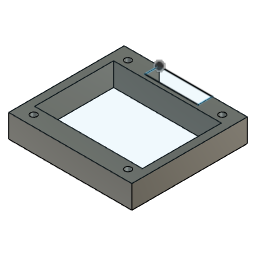
OLEDHolder (Autodesk Fusion 360 design; units mm, degrees)
Autodesk Fusion 360 part; units mm, degrees
sketch "Sketch1" plane through (0, 0, 0) normal (0, 0, 1) x (1, 0, 0)
  line L0 (16, 15) -> (-16, 15)
  line L1 (-16, 15) -> (-16, -15)
  line L2 (-16, -15) -> (16, -15)
  line L3 (16, -15) -> (16, 15)
  line L4 (16, 15) -> (-16, -15) construction
  line L5 (-16, 15) -> (16, -15) construction
  line L6 (14, 10.25) -> (-14, 10.25)
  line L7 (-14, 10.25) -> (-14, -10.25)
  line L8 (-14, -10.25) -> (14, -10.25)
  line L9 (14, -10.25) -> (14, 10.25)
  line L10 (14, 10.25) -> (-14, -10.25) construction
  line L11 (-14, 10.25) -> (14, -10.25) construction
  dimension "d1" = 32
  dimension "d2" = 30
  dimension "d3" = 28
  dimension "d4" = 20.5
  constraint horizontal L0
  constraint perpendicular L0 L1
  constraint parallel L0 L2
  constraint parallel L1 L3
  constraint coincident L4 origin
  constraint coincident L5 origin
  constraint horizontal L6
  constraint perpendicular L6 L7
  constraint parallel L6 L8
  constraint parallel L7 L9
  constraint coincident L10 origin
  constraint coincident L11 origin
  measures "d1" distance of L1.end L2.end
  measures "d2" distance of L0.end L1.end
  measures "d3" distance of L7.end L8.end
  measures "d4" distance of L6.end L7.end
extrude "Extrude1" add sketch "Sketch1" along normal blind 6
sketch "Sketch2" plane through (0, 0, 6) normal (0, 0, 1) x (-1, 0, 0)
  line L0 (-14, -10.25) -> (-14, 10.25)
  line L1 (-14, 10.25) -> (14, 10.25)
  line L2 (14, 10.25) -> (14, -10.25)
  line L3 (14, -10.25) -> (-14, -10.25)
  line L4 (-16, 15) -> (-16, -15)
  line L5 (-16, -15) -> (16, -15)
  line L6 (16, -15) -> (16, 15)
  line L7 (16, 15) -> (-16, 15)
  line L8 (6.895, -15) -> (-6.895, -15)
  line L9 (-6.895, -15) -> (-6.895, -11.3)
  line L10 (-6.895, -11.3) -> (6.895, -11.3)
  line L11 (6.895, -11.3) -> (6.895, -15)
  dimension "d7" = 13.79
  dimension "d8" = 3.7
  constraint horizontal L8
  constraint vertical L9
  constraint horizontal L10
  constraint vertical L11
  constraint coincident L5 L8.start
  measures "d7" distance of L8.start L8.end
  measures "d8" distance of L8.start L10.end
extrude "Extrude2" cut sketch "Sketch2" against normal blind 5 contours L5 L8 L9 L10 L11
sketch "Sketch3" plane through (0, 0, 6) normal (0, 0, 1) x (-1, 0, 0)
  line L0 (6.895, -11.3) -> (6.895, -15)
  line L1 (6.895, -15) -> (16, -15)
  line L2 (16, -15) -> (16, 15)
  line L3 (16, 15) -> (-16, 15)
  line L4 (-16, 15) -> (-16, -15)
  line L5 (-16, -15) -> (-6.895, -15)
  line L6 (-6.895, -15) -> (-6.895, -11.3)
  line L7 (-6.895, -11.3) -> (6.895, -11.3)
  line L8 (-14, -10.25) -> (-14, 10.25)
  line L9 (-14, 10.25) -> (14, 10.25)
  line L10 (14, 10.25) -> (14, -10.25)
  line L11 (14, -10.25) -> (-14, -10.25)
  line L12 (-13.75, -13.75) -> (13.75, -13.75)
  line L13 (13.75, -13.75) -> (13.75, 13.75)
  line L14 (13.75, 13.75) -> (-13.75, 13.75)
  line L15 (-13.75, 13.75) -> (-13.75, -13.75)
  line L16 (-13.75, -13.75) -> (13.75, 13.75) construction
  line L17 (13.75, -13.75) -> (-13.75, 13.75) construction
  line L18 (-13.75, -13.75) -> (-12.25, -13.75)
  line L19 (-12.25, -13.75) -> (-12.25, -12.25)
  line L20 (-13.75, -12.25) -> (-13.75, -13.75)
  circle A0 centre (-12.25, -12.25) radius 0.85
  line L21 (13.75, -13.75) -> (12.25, -13.75)
  line L22 (12.25, -13.75) -> (12.25, -12.25)
  line L23 (13.75, -12.25) -> (13.75, -13.75)
  circle A1 centre (12.25, -12.25) radius 0.85
  line L24 (13.75, 13.75) -> (12.25, 13.75)
  line L25 (12.25, 13.75) -> (12.25, 12.25)
  line L26 (13.75, 12.25) -> (13.75, 13.75)
  circle A2 centre (12.25, 12.25) radius 0.85
  line L27 (-13.75, 13.75) -> (-12.25, 13.75)
  line L28 (-12.25, 13.75) -> (-12.25, 12.25)
  line L29 (-13.75, 12.25) -> (-13.75, 13.75)
  circle A3 centre (-12.25, 12.25) radius 0.85
  dimension "d11" = 27.5
  dimension "d12" = 27.5
  dimension "d13" = 1.5
  dimension "d14" = 1.5
  dimension "d15" = 1.7
  dimension "d16" = 1.5
  dimension "d17" = 1.5
  dimension "d18" = 1.7
  dimension "d19" = 1.5
  dimension "d20" = 1.5
  dimension "d21" = 1.7
  dimension "d22" = 1.5
  dimension "d23" = 1.5
  dimension "d24" = 1.7
  constraint horizontal L12
  constraint perpendicular L12 L13
  constraint parallel L12 L14
  constraint parallel L13 L15
  constraint coincident L16 origin
  constraint coincident L17 origin
  constraint horizontal L18
  constraint vertical L19
  constraint vertical L20
  constraint coincident L19.end A0.centre
  constraint horizontal L21
  constraint vertical L22
  constraint vertical L23
  constraint coincident L22.end A1.centre
  constraint horizontal L24
  constraint vertical L25
  constraint vertical L26
  constraint coincident L25.end A2.centre
  constraint horizontal L27
  constraint vertical L28
  constraint vertical L29
  constraint coincident L28.end A3.centre
  measures "d11" distance of L13.end L14.end
  measures "d12" distance of L12.end L13.end
  measures "d13" distance of L12.start L18.end
  measures "d14" distance of L12.start L20.start
  measures "d15" diameter of A0
  measures "d16" distance of L12.end L21.end
  measures "d17" distance of L12.end L23.start
  measures "d18" diameter of A1
  measures "d19" distance of L13.end L24.end
  measures "d20" distance of L13.end L26.start
  measures "d21" diameter of A2
  measures "d22" distance of L14.end L27.end
  measures "d23" distance of L14.end L29.start
  measures "d24" diameter of A3
extrude "Extrude3" cut sketch "Sketch3" against normal blind 5 contours A0 | A1 | A2 | A3
